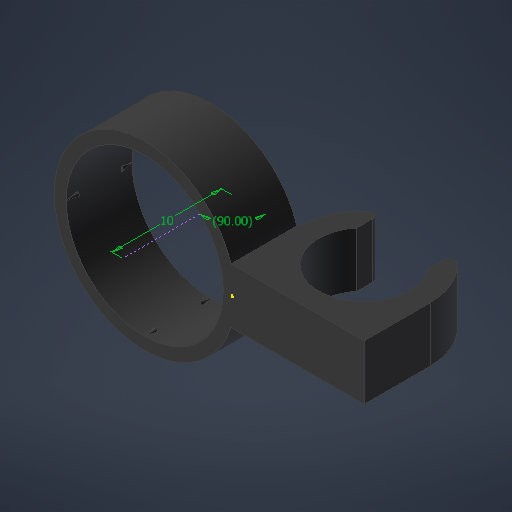
# Autodesk Inventor part: AgarreColganteCabina_v02
Saved by Autodesk Inventor 2026.1 (Build 301233020, 233B)
## iProperties
Created: 2025-11-02
Part Number: AgarreColganteCabina_v02
Material: Generic
Document SubType Name: Modeling
Designer: Tito Luyo Murata
Density: 1 g/cm^3
Appearance: Default
Author: Tito Luyo Murata
Autodesk Inventor part; units mm, degrees
ref_plane "YZ Plane" through (0, 0, 0) normal (1, 0, 0) x (0, 1, 0)
ref_plane "XZ Plane" through (0, 0, 0) normal (0, 1, 0) x (-1, 0, 0)
ref_plane "XY Plane" through (0, 0, 0) normal (0, 0, 1) x (1, 0, 0)
sketch "Sketch5" plane through (0, 0, 0) normal (0, 1, 0) x (-1, 0, 0)
  line L0 (0, 0) -> (-12, 0)
  line L1 (-12, 0) -> (-12, -12)
  line L2 (-12, -12) -> (0, -12)
  line L3 (0, -12) -> (0, 0)
  circle A0 centre (-6, -6) radius 4.15
  circle A1 centre (-6, -6) radius 6
  line L4 (-6, -6) -> (-6, -14) construction
  line L5 (-2.75, -8) -> (-9.25, -8)
  line L6 (-9.25, -8) -> (-9.25, -12)
  line L7 (-9.25, -12) -> (-2.75, -12)
  line L8 (-2.75, -12) -> (-2.75, -8)
  line L9 (-2.75, -8) -> (-9.25, -12) construction
  line L10 (-9.25, -8) -> (-2.75, -12) construction
  point P0 (-6, -10)
  point P1 (-12, -6)
  point P2 (-9.25, -11.0436)
  point P3 (-9.25, -8.5807)
  point P4 (-2.75, -8.5807)
  point P5 (-2.75, -11.0436)
  point P6 (0, -6)
  dimension "d10" = 12
  dimension "d11" = 12
  dimension "d12" = 8.3
  dimension "d13" = 12
  dimension "d14" = 8
  dimension "d15" = 6.5
  constraints: 22 end point, 4 parallel, 3 midpoint, 2 centre point, 2 horizontal, 2 perpendicular, 1 coincident, 1 point on line, 1 vertical
  measures "d10" distance of L2.end L1.end
  measures "d11" distance of L1.end L0.end
  measures "d12" diameter of A0
  measures "d13" diameter of A1
  measures "d14" distance of L4.start L4.end
  measures "d15" distance of L7.end L6.end
extrude "Extrusion3" add sketch "Sketch5" along normal blind 5 contours L3 A1 L0 | A1 L1 L0 | A1 L8 A0 L6 picked at (-9.6317, -9.9029)
fillet "Fillet1" radius 0.5 2 edges at (2.75, 2.5, -11.0436) (9.25, 2.5, -11.0436)
sketch "Sketch6" plane through (0, 0, 0) normal (0, 0, 1) x (1, 0, 0)
  circle A0 centre (-8, 2.5) radius 8.25
  line L0 (0, 0) -> (0, 5) projected
  line L1 (0, 5) -> (-0.5, 5)
  line L2 (-0.5, 5) -> (-0.5, 0)
  line L3 (-0.5, 0) -> (0, 0)
  line L4 (0, 0) -> (0, 5)
  circle A1 centre (-8, 2.5) radius 7.15
  point P0 (-0.1379, 0)
  point P1 (-0.1379, 5)
  dimension "d19" = 16.5
  dimension "d20" = 0.5
  dimension "d21" = 5
  dimension "d22" = 14.3
  constraints: 8 end point, 2 centre point, 2 parallel, 1 coincident, 1 horizontal, 1 perpendicular
  measures "d19" diameter of A0
  measures "d20" distance of L3.end L2.end
  measures "d21" distance of L2.end L1.end
  measures "d22" diameter of A1
extrude "Extrusion4" add sketch "Sketch6" against normal blind 6 contours L0 A0 L3 L2 L1 | A0 L1 L0 | L0 L3 A0 | L1 L2 L3 A0
ref_plane "Work Plane1" through (0, 2.5, 0) normal (0, -1, 0) x (1, 0, 0)
sketch "Sketch7" plane through (0, 2.5, 0) normal (0, -1, 0) x (1, 0, 0)
  line L0 (-0.85, -6) -> (-15.15, -6) projected
  line L1 (-0.85, -6) -> (-0.85, -5)
  line L2 (-0.85, -6) -> (0.15, -6) construction
  line L3 (-0.85, -5) -> (-1.05, -5)
  line L4 (12, 0) -> (-0.1379, 0) projected
  line L5 (-0.85, -5) -> (-0.65, -5) construction
  line L6 (-1.05, -5) -> (-0.85, -6)
  line L7 (-0.85, -6) -> (-0.85, 0) construction
  point P0 (0, 0)
  dimension "d25" = 1
  dimension "d26" = 90
  dimension "d27" = 0.2
  dimension "d28" = 180
  constraints: 12 end point, 2 equal length, 2 horizontal, 1 parallel, 1 perpendicular
  measures "d25" distance of L0.start L1.end
  measures "d26" angle of L2 L1
  measures "d27" distance of L1.end L3.end
  measures "d28" angle of L3 L5
revolve "Revolution1" add sketch "Sketch7" angle 360 about axis through (-0.85, 2.5, -6) along (0, 0, 1)
sketch "Sketch8" plane through (0, 2.5, 0) normal (0, -1, 0) x (1, 0, 0)
  line L0 (-8, -8) -> (-8, 2) construction
  line L1 (-8, -8) -> (2, -8) construction
  point P0 (0, 0)
  dimension "d30" = 10
  dimension "d31" = 90
  constraints: 4 end point, 1 horizontal, 1 perpendicular, 1 vertical
  measures "d30" distance of L0.start L0.end
  measures "d31" angle of L1 L0
pattern_circular "Circular Pattern1" count 4 over 360 about axis through (-8, 2.5, 0) along (0, 0, -1) of "Revolution1"
ref_plane "Work Plane2" through (0, 0, -3) normal (0, 0, -1) x (-1, 0, 0)
mirror "Mirror1" about plane through (0, 0, -3) normal (0, 0, -1) of "Revolution1", "Circular Pattern1"
equation "\"tol\" = 0.3"
body "Solid2"
